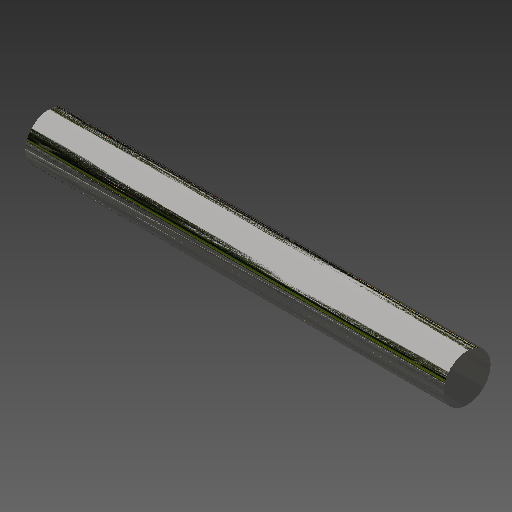
# Autodesk Inventor part: 3d_LM-Welding_Tooling -  Guide Pin
Saved by Autodesk Inventor 2018.3 (Build 223284000, 284)
## iProperties
Created: 2026-01-20
Part Number: 3d_LM-Welding_Tooling -  Guide Pin
Material: 304 Stainless Steel
Document SubType Name: Modeling
Designer: aca6
Density: 8 g/cm^3
Appearance: N/A - Machined Stainless Steel
Manufacturer-1: {"Name": "FABORY SPAIN S.L.U.", "PartNumber": "3d_Welding_Tooling -  Guide Pin", "Link": "https://www.fabory.com/es/pasador-din-7-m6-acero-inoxidable-%28inox%29-a1-a2-2x18mm-sku/p/51580020018"}
Manufacturer-2: {"Name": "", "PartNumber": "", "Link": ""}
Manufacturer-3: {"Name": "", "PartNumber": "", "Link": ""}
Manufacturer-4: {"Name": "", "PartNumber": "", "Link": ""}
Manufacturer-5: {"Name": "", "PartNumber": "", "Link": ""}
Provider-1: {"Name": "FABORY SPAIN S.L.U.", "PartNumber": "3d_Welding_Tooling -  Guide Pin", "Link": "https://www.fabory.com/es/pasador-din-7-m6-acero-inoxidable-%28inox%29-a1-a2-2x18mm-sku/p/51580020018"}
Provider-2: {"Name": "", "PartNumber": "", "Link": ""}
Provider-3: {"Name": "", "PartNumber": "", "Link": ""}
Provider-4: {"Name": "", "PartNumber": "", "Link": ""}
Provider-5: {"Name": "", "PartNumber": "", "Link": ""}
Author: aca6
Autodesk Inventor part; units mm, degrees
ref_plane "YZ Plane" through (0, 0, 0) normal (1, 0, 0) x (0, 1, 0)
ref_plane "XZ Plane" through (0, 0, 0) normal (0, 1, 0) x (-1, 0, 0)
ref_plane "XY Plane" through (0, 0, 0) normal (0, 0, 1) x (1, 0, 0)
sketch "Sketch2" plane through (0, 0, 0) normal (0, 0, 1) x (1, 0, 0)
  line L0 (-9, 1) -> (8.8284, 1)
  line L1 (8.8284, 1) -> (8.8284, 0)
  line L2 (8.8284, 0) -> (-9.1716, 0)
  line L3 (-9, 0) -> (-9, 1)
  line L4 (0, 0) -> (3.6926, 0)
  line L5 (8.8284, 0) -> (9.1716, 0)
  arc A0 (-9, 1) -> (-9, -1) centre (-6.1716, 0) ccw
  line L6 (0, 0) -> (0, 0.5) construction
  dimension "d3" = 1
  dimension "d7" = 2
  dimension "d8" = 3
  dimension "d11" = 18
  constraints: 14 end point, 3 horizontal, 3 point on circle, 3 point on line, 3 vertical, 2 perpendicular, 1 centre point, 1 symmetric about line, 2 other
  measures "d3" distance of L0.end L1.end
  measures "d7" distance of L0.start A0.end
  measures "d8" radius of A0
  measures "d11" distance from line of L2.end L1
revolve "Revolution1" add sketch "Sketch2" angle 360 about axis through (0, 0, 0) along (1, 0, 0)
body "Solid2"
